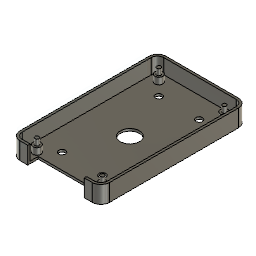
wall-mount-touch-display (Autodesk Fusion 360 design; units mm, degrees)
Autodesk Fusion 360 part; units mm, degrees
sketch "Skizze2" plane through (0, 0, 0) normal (0, 0, 1) x (1, 0, 0)
  line L0 (0, 0) -> (50, 0)
  line L1 (50, 0) -> (50, 86)
  line L2 (50, 86) -> (0, 86)
  line L3 (0, 86) -> (0, 0)
  circle A0 centre (4.2, 5.1408) radius 1.25
  line L4 (25, 86) -> (25, 0) construction
  line L5 (0, 40) -> (50, 40) construction
  circle A1 centre (4.2, 5.1408) radius 2.5
  circle A2 centre (45.8, 5.1408) radius 1.25
  circle A3 centre (45.8, 5.1408) radius 2.5
  circle A4 centre (4.2, 82.6408) radius 1.25
  circle A5 centre (4.2, 82.6408) radius 2.5
  circle A6 centre (45.8, 82.6408) radius 2.5
  circle A7 centre (45.8, 82.6408) radius 1.25
  line L6 (43, 0) -> (7, 0)
  line L7 (7, 0) -> (7, 3.137)
  line L8 (7, 3.137) -> (43, 3.137)
  line L9 (43, 3.137) -> (43, 0)
  line L10 (43, 0) -> (7, 3.137) construction
  line L11 (7, 0) -> (43, 3.137) construction
  line L12 (50, 10) -> (0, 10) construction
  line L13 (0, 79.4) -> (50, 79.4) construction
  line L14 (0, 10) -> (0, 79.4) construction
  line L15 (0, 44.7) -> (50, 44.7) construction
  line L16 (2, -2) -> (48, -2)
  line L17 (52, 2) -> (52, 84)
  line L18 (48, 88) -> (2, 88)
  line L19 (-2, 84) -> (-2, 2)
  arc A8 (52, 84) -> (48, 88) centre (48, 84) ccw
  arc A9 (2, 88) -> (-2, 84) centre (2, 84) ccw
  arc A10 (-2, 2) -> (2, -2) centre (2, 2) ccw
  arc A11 (48, -2) -> (52, 2) centre (48, 2) ccw
  line L20 (-3.5, 84) -> (-3.5, 2)
  arc A12 (-3.5, 2) -> (2, -3.5) centre (2, 2) ccw
  line L21 (2, -3.5) -> (48, -3.5)
  arc A13 (48, -3.5) -> (53.5, 2) centre (48, 2) ccw
  line L22 (53.5, 2) -> (53.5, 84)
  arc A14 (53.5, 84) -> (48, 89.5) centre (48, 84) ccw
  line L23 (48, 89.5) -> (2, 89.5)
  arc A15 (2, 89.5) -> (-3.5, 84) centre (2, 84) ccw
  line L24 (7, 0) -> (7, -3.5)
  line L25 (43, 0) -> (43, -3.5)
  point P0 (25, 1.5685)
  dimension "d3" = 50
  dimension "d4" = 86
  dimension "d5" = 2.5
  dimension "d6" = 5
  dimension "d7" = 2.5
  dimension "d8" = 5
  dimension "d10" = 4
  dimension "d11" = 1.5
  dimension "d108" = 20.8
  dimension "d109" = 77.5
  dimension "d110" = 20.8
  constraint horizontal L0
  constraint vertical L1
  constraint horizontal L2
  constraint vertical L3
  constraint coincident L0.start L3.end
  constraint midpoint L2 L4.start
  constraint midpoint L0 L4.end
  constraint coincident L3 L5.start
  constraint coincident L1 L5.end
  constraint perpendicular L1 L5
  constraint concentric A0 A1
  constraint symmetric A0 L4 A2
  constraint symmetric L4 A1 A3
  constraint concentric A4 A5
  constraint symmetric L4 A4 A7
  constraint symmetric L4 A5 A6
  constraint horizontal L6
  constraint perpendicular L6 L7
  constraint parallel L6 L8
  constraint parallel L7 L9
  constraint coincident L10 P0
  constraint coincident L11 P0
  constraint coincident L0 L6.start
  constraint coincident L4 P0
  constraint coincident L1 L12.start
  constraint coincident L3 L12.end
  constraint perpendicular L3 L12
  constraint coincident L3 L13.start
  constraint coincident L1 L13.end
  constraint perpendicular L1 L13
  constraint midpoint L14 L15.start
  constraint coincident L1 L15.end
  constraint perpendicular L1 L15
  constraint tangent L17 A8
  constraint tangent L18 A8
  constraint tangent L18 A9
  constraint tangent L19 A9
  constraint equal A8 A9
  constraint tangent L16 A10
  constraint tangent L19 A10
  constraint equal A8 A10
  constraint tangent L16 A11
  constraint tangent L17 A11
  constraint equal A8 A11
  constraint coincident L21 L24.end
  constraint perpendicular L21 L24
  constraint coincident L21 L25.end
  constraint perpendicular L21 L25
  measures "d3" distance of L0.start L0.end
  measures "d4" distance of L0.start L2.end
  measures "d5" diameter of A0
  measures "d6" diameter of A1
  measures "d7" diameter of A4
  measures "d8" diameter of A5
  measures "d10" radius of A8
  measures "d108" distance of L4 A6.centre
  measures "d109" vertical distance of A2.centre A6.centre
  measures "d110" distance of L4 A2.centre
extrude "Extrusion1" add sketch "Skizze2" along normal blind 8.6 contours L16 L17 L18 L19 A8 A9 A10 A11 L20 A12 L21 A13 L22 A14 L23 A15 L24 L25 makes body 1
extrude "Extrusion2" add sketch "Skizze2" against normal blind 1.5 contours L0 L1 L2 L3 L7 L8 L9 | L0 L1 L2 L3 L16 L17 L18 L19 A8 A9 A10 A11 L24 L25 | L16 L17 L18 L19 A8 A9 A10 A11 L20 A12 L21 A13 L22 A14 L23 A15 L24 L25 | A0 | A1 | A2 | A3 | A4 | A5 | A6 | A7 bodies 1
extrude "Extrusion3" add sketch "Skizze2" along normal blind 4.2 contours A1 | A3 | A5 | A6 bodies 1
extrude "Extrusion4" add sketch "Skizze2" along normal blind 4.2 contours A0 | A2 | A4 | A7 bodies 1
sketch "Skizze3" plane through (0, 0, 0) normal (0, 0, 1) x (1, 0, 0)
  arc A0 (2, 89.5) -> (-3.5, 84) centre (2, 84) ccw
  line L0 (-3.5, 84) -> (-3.5, 2)
  arc A1 (-3.5, 2) -> (2, -3.5) centre (2, 2) ccw
  line L1 (2, -3.5) -> (48, -3.5)
  arc A2 (48, -3.5) -> (53.5, 2) centre (48, 2) ccw
  line L2 (53.5, 2) -> (53.5, 84)
  arc A3 (53.5, 84) -> (48, 89.5) centre (48, 84) ccw
  line L3 (48, 89.5) -> (2, 89.5)
  circle A4 centre (4.2, 82.6408) radius 2.5
  circle A5 centre (45.8, 82.6408) radius 2.5
  circle A6 centre (45.8, 5.1408) radius 2.5
  circle A7 centre (4.2, 5.1408) radius 2.5
  arc A8 (-3.55, 2) -> (2, -3.55) centre (2, 2) ccw
  line L4 (2, -3.55) -> (48, -3.55)
  arc A9 (48, -3.55) -> (53.55, 2) centre (48, 2) ccw
  line L5 (53.55, 2) -> (53.55, 84)
  arc A10 (53.55, 84) -> (48, 89.55) centre (48, 84) ccw
  line L6 (48, 89.55) -> (2, 89.55)
  arc A11 (2, 89.55) -> (-3.55, 84) centre (2, 84) ccw
  line L7 (-3.55, 84) -> (-3.55, 2)
  line L8 (48, 91.05) -> (2, 91.05)
  arc A12 (2, 91.05) -> (-5.05, 84) centre (2, 84) ccw
  line L9 (-5.05, 84) -> (-5.05, 2)
  arc A13 (-5.05, 2) -> (2, -5.05) centre (2, 2) ccw
  line L10 (2, -5.05) -> (48, -5.05)
  arc A14 (48, -5.05) -> (55.05, 2) centre (48, 2) ccw
  line L11 (55.05, 2) -> (55.05, 84)
  arc A15 (55.05, 84) -> (48, 91.05) centre (48, 84) ccw
  dimension "d26" = 0.05
  dimension "d27" = 1.55
extrude "Extrusion6" add sketch "Skizze3" against normal blind 1.8 separate body contours L8 A12 L9 A13 L10 A14 L11 A15 makes body 2
extrude "Extrusion7" add sketch "Skizze3" along normal blind 8.6 contours L8 A12 L9 A13 L10 A14 L11 A15 bodies 2
sketch "Skizze4" plane through (0, 0, 8.6) normal (0, 0, 1) x (-1, 0, 0)
  line L0 (3.55, -2) -> (3.55, -84)
  arc A0 (-2, -89.55) -> (3.55, -84) centre (-2, -84) ccw
  line L1 (-2, -89.55) -> (-48, -89.55)
  arc A1 (-53.55, -84) -> (-48, -89.55) centre (-48, -84) ccw
  line L2 (-53.55, -84) -> (-53.55, -2)
  arc A2 (-48, 3.55) -> (-53.55, -2) centre (-48, -2) ccw
  line L3 (-48, 3.55) -> (-2, 3.55)
  arc A3 (3.55, -2) -> (-2, 3.55) centre (-2, -2) ccw
  arc A4 (-55.05, -84) -> (-48, -91.05) centre (-48, -84) ccw
  line L4 (-48, -91.05) -> (-2, -91.05)
  arc A5 (-2, -91.05) -> (5.05, -84) centre (-2, -84) ccw
  line L5 (5.05, -84) -> (5.05, -2)
  arc A6 (5.05, -2) -> (-2, 5.05) centre (-2, -2) ccw
  line L6 (-2, 5.05) -> (-48, 5.05)
  arc A7 (-48, 5.05) -> (-55.05, -2) centre (-48, -2) ccw
  line L7 (-55.05, -2) -> (-55.05, -84)
  line L8 (5.05, -84) -> (5.05, -2)
  arc A8 (-2, -91.05) -> (5.05, -84) centre (-2, -84) ccw
  line L9 (-48, -91.05) -> (-2, -91.05)
  arc A9 (-55.05, -84) -> (-48, -91.05) centre (-48, -84) ccw
  line L10 (-55.05, -2) -> (-55.05, -84)
  arc A10 (-48, 5.05) -> (-55.05, -2) centre (-48, -2) ccw
  line L11 (-2, 5.05) -> (-48, 5.05)
  arc A11 (5.05, -2) -> (-2, 5.05) centre (-2, -2) ccw
  line L12 (0, -79.4) -> (-50, -79.4) construction
  line L13 (-50, -10) -> (0, -10) construction
  circle A12 centre (-4.2, -82.6408) radius 2.5
  circle A13 centre (-45.8, -82.6408) radius 2.5
  circle A14 centre (-45.8, -82.6408) radius 2.5
  circle A15 centre (-45.8, -5.1408) radius 2.5
  circle A16 centre (-45.8, -5.1408) radius 2.5
  circle A17 centre (-4.2, -5.1408) radius 2.5
  line L14 (0, -79.4) -> (0, -10) construction
  line L15 (-50, -79.4) -> (-50, -10) construction
  line L16 (0, -77.4) -> (-50, -77.4) construction
  line L17 (-50, -17.7) -> (0, -17.7) construction
  line L18 (-48, -79.4) -> (-48, -10) construction
  line L19 (-2, -79.4) -> (-2, -10) construction
  line L20 (-2, -77.4) -> (-48, -77.4)
  line L21 (-48, -77.4) -> (-48, -17.7)
  line L22 (-48, -17.7) -> (-2, -17.7)
  line L23 (-2, -17.7) -> (-2, -77.4)
  circle A18 centre (-45.8, -82.6408) radius 1.4
  circle A19 centre (-4.2, -82.6408) radius 1.4
  circle A20 centre (-45.8, -5.1408) radius 1.4
  circle A21 centre (-4.2, -5.1408) radius 1.4
  dimension "d32" = 2
  dimension "d33" = 7.7
  dimension "d34" = 2
  dimension "d35" = -2
  dimension "d44" = 2.8
  dimension "d45" = 2.8
  dimension "d46" = 2.8
  dimension "d47" = 2.8
  constraint coincident L12.start L14.start
  constraint coincident L13.end L14.end
  constraint coincident L12.end L15.start
  constraint coincident L13.start L15.end
  constraint horizontal L20
  constraint vertical L21
  constraint horizontal L22
  constraint vertical L23
  constraint coincident L18 L21.end
  constraint coincident L17 L21.end
  constraint coincident L19 L20.start
  constraint coincident L16 L20.start
  measures "d44" diameter of A18
  measures "d45" diameter of A19
  measures "d46" diameter of A20
  measures "d47" diameter of A21
extrude "Extrusion8" add sketch "Skizze4" along normal blind 1 contours L0 A0 L1 A1 L2 A2 L3 A3 | A4 L4 A5 L5 A6 L6 A7 L7 L8 A8 L9 A9 L10 A10 L11 A11 | A12 | A13 A14 | A15 A16 | A17 | A18 | A19 | A20 | A21 bodies 2
extrude "Extrusion9" add sketch "Skizze4" against normal blind 2.4 contours A12 | A13 A14 | A15 A16 | A17 | A18 | A19 | A20 | A21 bodies 2
sketch "Skizze5" plane through (0, 0, 9.6) normal (0, 0, 1) x (-1, 0, 0)
  line L0 (-48, -17.7) -> (-2, -17.7)
  line L1 (-2, -17.7) -> (-2, -77.4)
  line L2 (-2, -77.4) -> (-48, -77.4)
  line L3 (-48, -77.4) -> (-48, -17.7)
  arc A0 (5.05, -2) -> (-2, 5.05) centre (-2, -2) ccw
  line L4 (-2, 5.05) -> (-48, 5.05)
  arc A1 (-48, 5.05) -> (-55.05, -2) centre (-48, -2) ccw
  line L5 (-55.05, -2) -> (-55.05, -84)
  arc A2 (-55.05, -84) -> (-48, -91.05) centre (-48, -84) ccw
  line L6 (-48, -91.05) -> (-2, -91.05)
  arc A3 (-2, -91.05) -> (5.05, -84) centre (-2, -84) ccw
  line L7 (5.05, -84) -> (5.05, -2)
  line L8 (4.05, -84) -> (4.05, -2)
  arc A4 (4.05, -2) -> (-2, 4.05) centre (-2, -2) ccw
  line L9 (-2, 4.05) -> (-48, 4.05)
  arc A5 (-48, 4.05) -> (-54.05, -2) centre (-48, -2) ccw
  line L10 (-54.05, -2) -> (-54.05, -84)
  arc A6 (-54.05, -84) -> (-48, -90.05) centre (-48, -84) ccw
  line L11 (-48, -90.05) -> (-2, -90.05)
  arc A7 (-2, -90.05) -> (4.05, -84) centre (-2, -84) ccw
  line L12 (3.95, -84) -> (3.95, -2)
  arc A8 (3.95, -2) -> (-2, 3.95) centre (-2, -2) ccw
  line L13 (-2, 3.95) -> (-48, 3.95)
  arc A9 (-48, 3.95) -> (-53.95, -2) centre (-48, -2) ccw
  line L14 (-53.95, -2) -> (-53.95, -84)
  arc A10 (-53.95, -84) -> (-48, -89.95) centre (-48, -84) ccw
  line L15 (-48, -89.95) -> (-2, -89.95)
  arc A11 (-2, -89.95) -> (3.95, -84) centre (-2, -84) ccw
  dimension "d40" = -1
  dimension "d41" = -1.1
extrude "Extrusion10" cut sketch "Skizze5" against normal blind 0.1 contours L8 A4 L9 A5 L10 A6 L11 A7 bodies 2
sketch "Skizze6" plane through (0, 0, -1.5) normal (0, 0, -1) x (1, 0, 0)
  line L0 (7, -3.137) -> (7, 3.5)
  line L1 (7, 3.5) -> (2, 3.5)
  arc A0 (2, 3.5) -> (-3.5, -2) centre (2, -2) ccw
  line L2 (-3.5, -2) -> (-3.5, -84)
  arc A1 (-3.5, -84) -> (2, -89.5) centre (2, -84) ccw
  line L3 (2, -89.5) -> (48, -89.5)
  arc A2 (48, -89.5) -> (53.5, -84) centre (48, -84) ccw
  line L4 (53.5, -84) -> (53.5, -2)
  arc A3 (53.5, -2) -> (48, 3.5) centre (48, -2) ccw
  line L5 (48, 3.5) -> (43, 3.5)
  line L6 (43, 3.5) -> (43, -3.137)
  line L7 (43, -3.137) -> (7, -3.137)
  line L8 (2, 3.55) -> (48, 3.55)
  arc A4 (2, 3.55) -> (-3.55, -2) centre (2, -2) ccw
  arc A5 (53.55, -2) -> (48, 3.55) centre (48, -2) ccw
  line L9 (53.55, -2) -> (53.55, -84)
  arc A6 (48, -89.55) -> (53.55, -84) centre (48, -84) ccw
  line L10 (48, -89.55) -> (2, -89.55)
  arc A7 (-3.55, -84) -> (2, -89.55) centre (2, -84) ccw
  line L11 (-3.55, -84) -> (-3.55, -2)
  line L12 (25, 3.55) -> (25, -89.55) construction
  line L13 (-3.55, -43) -> (53.5, -43) construction
  line L14 (37, -79) -> (13, -79)
  line L15 (13, -79) -> (13, -7)
  line L16 (13, -7) -> (37, -7)
  line L17 (37, -7) -> (37, -79)
  line L18 (37, -79) -> (13, -7) construction
  line L19 (13, -79) -> (37, -7) construction
  circle A8 centre (28, -35) radius 3
  point P0 (25, -43)
  dimension "d49" = 24
  dimension "d121" = 6
  constraint midpoint L8 L12.start
  constraint midpoint L10 L12.end
  constraint midpoint L11 L13.start
  constraint midpoint L4 L13.end
  constraint horizontal L14
  constraint perpendicular L14 L15
  constraint parallel L14 L16
  constraint parallel L15 L17
  constraint coincident L18 P0
  constraint coincident L19 P0
  constraint midpoint L12 P0
  measures "d49" distance of L15.end L16.end
  measures "d121" diameter of A8
extrude "Extrusion11" add sketch "Skizze6" along normal blind 22 contours L14 L15 L16 L17 | A8 bodies 1
sketch "Skizze7" plane through (0, 79, 0) normal (0, 1, 0) x (-1, 0, 0)
  line L0 (-13, -1.5) -> (-37, -1.5)
  line L1 (-37, -1.5) -> (-37, -23.5)
  line L2 (-37, -23.5) -> (-13, -23.5)
  line L3 (-13, -23.5) -> (-13, -1.5)
  line L4 (-25, -23.5) -> (-25, -1.5) construction
  circle A0 centre (-25, -17) radius 12
  dimension "d52" = 24
  constraint midpoint L2 L4.start
  constraint midpoint L0 L4.end
  constraint coincident L4 A0.centre
  measures "d52" diameter of A0
extrude "Extrusion12" cut 1 faces at (21, 31, -23.5) along direction (0, 0, 1) blind 7 on bodies 1 bodies 1
fillet "Abrundung1" radius 12 1 edges at (25, 79, -16.5) on bodies 1
fillet "Abrundung2" radius 12 1 edges at (25, 7, -16.5) on bodies 1
extrude "Extrusion13" cut sketch "Skizze7" against normal blind 79 contours L2 A0 | L2 A0 bodies 1
sketch "Skizze16" plane through (0, 0, 0) normal (0, 0, 1) x (1, 0, 0)
  line L0 (37, 61) -> (13, 61)
  line L1 (13, 61) -> (13, 65)
  line L2 (13, 65) -> (37, 65)
  line L3 (37, 65) -> (37, 61)
  line L4 (37, 61) -> (13, 65) construction
  line L5 (13, 61) -> (37, 65) construction
  line L6 (37, 21) -> (13, 21)
  line L7 (13, 21) -> (13, 25)
  line L8 (13, 25) -> (37, 25)
  line L9 (37, 25) -> (37, 21)
  line L10 (37, 21) -> (13, 25) construction
  line L11 (13, 21) -> (37, 25) construction
  circle A0 centre (28, 35) radius 3
  line L12 (28, 38) -> (34, 38)
  line L13 (34, 38) -> (34, 32)
  line L14 (34, 32) -> (28, 32)
  line L15 (28, 32) -> (28, 38)
  line L16 (28, 38) -> (16, 38)
  line L17 (16, 38) -> (16, 32)
  line L18 (16, 32) -> (28, 32)
  line L19 (28, 32) -> (28, 38)
  point P0 (25, 63)
  point P1 (25, 23)
  constraint horizontal L0
  constraint perpendicular L0 L1
  constraint parallel L0 L2
  constraint parallel L1 L3
  constraint coincident L4 P0
  constraint coincident L5 P0
  constraint horizontal L6
  constraint perpendicular L6 L7
  constraint parallel L6 L8
  constraint parallel L7 L9
  constraint coincident L10 P1
  constraint coincident L11 P1
  constraint horizontal L12
  constraint vertical L13
  constraint horizontal L14
  constraint vertical L15
  constraint coincident A0 L12.start
  constraint horizontal L16
  constraint vertical L17
  constraint horizontal L18
  constraint vertical L19
extrude "Extrusion25" add 1 faces at (-3, 56.6667, 8.6) along direction (0, 0, 1) blind 0.9 on bodies 1 bodies 1
move_body "Verschieben1" bodies 2 to x (1, 0, 0) y (0, 1, 0) z (0, 0, 1) at (0, 0, 0.9)
extrude "Extrusion26" add 1 faces at (54.55, 29.3333, -0.9) along direction (0, 0, -1) blind 0.9 on bodies 2 bodies 2
extrude "Extrusion27" add sketch "Skizze2" along normal blind 8 contours A0 | A2 | A4 | A7 bodies 1
extrude "Extrusion28" add sketch "Skizze4" along normal blind 1 contours A12 | A13 A14 | A15 A16 | A17 bodies 2
extrude "Extrusion29" add sketch "Skizze4" against normal blind 2.8 contours A12 | A13 A14 | A15 A16 | A17 bodies 2
sketch "Skizze17" plane through (0, 0, 0) normal (0, 0, 1) x (1, 0, 0)
  line L0 (17, 32, -33) -> (33, 32, -33)
  line L1 (33, 32, -33) -> (33, 38, -33)
  line L2 (33, 38, -33) -> (17, 38, -33)
  line L3 (17, 38, -33) -> (17, 32, -33)
extrude "Extrusion34" cut 4 faces at (3.9935, 4.8544, 7.1) (3.9667, 82.2367, 7.1) (45.5667, 83.045, 7.1) (46.4103, 4.7622, 7.1) along direction (0, 0, 1) blind 1.5 on bodies 2 bodies 2
copy_body "Körper->Berechn1" bodies 1 removing the originals makes body 3 in component "Inner Body"
copy_body "Körper->Berechn2" bodies 2 removing the originals makes body 4 in component "Outer Body"
sketch "Skizze18" plane through (0, 0, 0) normal (0, 1, 0) x (1, 0, 0)
sketch "Skizze19" plane through (-5.05, 0, 0) normal (-1, 0, 0) x (0, -1, 0)
  line L0 (-84, 10.5) -> (-84, -1.8)
  line L1 (-84, -1.8) -> (-2, -1.8)
  line L2 (-2, -1.8) -> (-2, 10.5)
  line L3 (-2, 10.5) -> (-84, 10.5)
delete_face "Fläche löschen1" 1 faces at (37, 35, -6.5) on bodies 3 in component "Inner Body"
sketch "Skizze20" plane through (0, 0, 0) normal (0, 0, 1) x (-1, 0, 0)
  circle A0 centre (-4.2, -82.6408) radius 2.5
  circle A1 centre (-45.8, -82.6408) radius 2.5
  line L0 (-2, 2) -> (-7, 2)
  line L1 (-7, 2) -> (-7, -3.137)
  line L2 (-7, -3.137) -> (-43, -3.137)
  line L3 (-43, -3.137) -> (-43, 2)
  line L4 (-43, 2) -> (-48, 2)
  arc A2 (-48, 2) -> (-52, -2) centre (-48, -2) ccw
  line L5 (-52, -2) -> (-52, -84)
  arc A3 (-52, -84) -> (-48, -88) centre (-48, -84) ccw
  line L6 (-48, -88) -> (-2, -88)
  arc A4 (-2, -88) -> (2, -84) centre (-2, -84) ccw
  line L7 (2, -84) -> (2, -2)
  arc A5 (2, -2) -> (-2, 2) centre (-2, -2) ccw
  circle A6 centre (-4.2, -5.1408) radius 2.5
  circle A7 centre (-45.8, -5.1408) radius 2.5
  circle A8 centre (-25, -43.4454) radius 6
  line L8 (-4.2, -82.6408) -> (-12.2, -82.6408) construction
  line L9 (-12.2, -82.6408) -> (-12.2, -74.6408) construction
  circle A9 centre (-12.2, -74.6408) radius 2.1
  line L10 (-25, -88) -> (-25, -5.1408) construction
  line L11 (-4.2, -5.1408) -> (-12.2, -5.1408) construction
  line L12 (-12.2, -5.1408) -> (-12.2, -13.1408) construction
  circle A10 centre (-12.2, -13.1408) radius 2.1
  circle A11 centre (-37.8, -13.1408) radius 2.1
  circle A12 centre (-37.8, -74.6408) radius 2.1
  dimension "d152" = 12
  dimension "d155" = 8
  dimension "d156" = 8
  dimension "d157" = 4.2
  dimension "d158" = 8
  dimension "d159" = 8
  dimension "d160" = 4.2
  dimension "d151" = 4.2
  constraint coincident A0.centre L8.start
  constraint perpendicular L8 L9
  constraint coincident L9.end A9.centre
  constraint midpoint L6 L10.start
  constraint perpendicular L2 L10
  constraint coincident A6.centre L11.start
  constraint perpendicular L7 L11
  constraint perpendicular L11 L12
  constraint coincident L12.end A10.centre
  constraint symmetric A9 L10 A12
  constraint symmetric L10 A10 A11
  measures "d152" diameter of A8
  measures "d155" distance of A0.centre L8.end
  measures "d156" distance of L8.end L9.end
  measures "d157" diameter of A9
  measures "d158" distance of A6.centre L11.end
  measures "d159" distance of L11.end L12.end
  measures "d160" diameter of A10
extrude "Extrusion2'" cut sketch "Skizze20" against normal blind 5 contours A8 | A9 | A10 | A11 | A12 bodies 3 in component "Inner Body"
component "Case" placed x (1, 0, 0) y (0, 1, 0) z (0, 0, 1) at (0, 0, 0)
component "Inner Body" placed x (1, 0, 0) y (0, 1, 0) z (0, 0, 1) at (0, 0, 0) in component "Case"
component "Outer Body" placed x (1, 0, 0) y (0, 1, 0) z (0, 0, 1) at (0, 0, 0) in component "Case"
named bodies: "Inner Body", "Outer Body"
